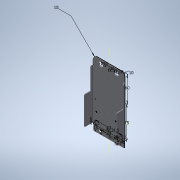
# Autodesk Inventor part: Enclosure_Base
Saved by Autodesk Inventor 2022 (Build 260153000, 153)
## iProperties
Created: 2023-10-31
Part Number: Enclosure_Base
Material: Generic
Document SubType Name: Sheet Metal
Designer: Baaij
Density: 1 g/cm^3
Sheet Metal Rule: Default_mm
Appearance: Default
Flat Pattern Width: 15 cm
Flat Pattern Length: 11.0786 cm
Flat Pattern Area: 166.179 cm^2
Sheet Metal Width: 150.000 mm
Sheet Metal Length: 110.786 mm
Sheet Metal Area: 16617.876 mm^2
Author: Baaij
Autodesk Inventor part; units mm, degrees
note: some values were not read from the file. Chosen so that the rebuilt part matches the saved one: relief shape of "Plate7"; flange form of "Plate6"; flange form of "Plate7"; relief shape of "Plate6".
ref_plane "YZ Plane" through (0, 0, 0) normal (1, 0, 0) x (0, 1, 0)
ref_plane "XZ Plane" through (0, 0, 0) normal (0, 1, 0) x (-1, 0, 0)
ref_plane "XY Plane" through (0, 0, 0) normal (0, 0, 1) x (1, 0, 0)
sketch "Sketch_base" plane through (0, 0, 0) normal (0, 0, 1) x (1, 0, 0)
  line L0 (0, 129.9853) -> (0, -82.9142) construction
  line L1 (-53.9995, 0) -> (53.9995, 0) construction
  line L2 (-36.5, 37.5) -> (36.5, 37.5)
  line L3 (36.5, 37.5) -> (36.5, -37.5)
  line L4 (36.5, -37.5) -> (-36.5, -37.5)
  line L5 (-36.5, -37.5) -> (-36.5, 37.5)
  line L6 (-36.5, 37.5) -> (36.5, -37.5) construction
  line L7 (36.5, 37.5) -> (-36.5, -37.5) construction
  line L8 (-35, -37.5) -> (35, -37.5)
  line L9 (35, -37.5) -> (35, -52.5)
  line L10 (35, -52.5) -> (-35, -52.5)
  line L11 (-35, -52.5) -> (-35, -37.5)
  line L12 (-35, -37.5) -> (35, -52.5) construction
  line L13 (35, -37.5) -> (-35, -52.5) construction
  line L14 (-26.5, 97.5) -> (26.5, 97.5)
  line L15 (36.5, 87.5) -> (36.5, 37.5)
  line L16 (36.5, 37.5) -> (-36.5, 37.5)
  line L17 (-36.5, 37.5) -> (-36.5, 87.5)
  line L18 (-36.5, 97.5) -> (36.5, 37.5) construction
  line L19 (36.5, 97.5) -> (-36.5, 37.5) construction
  arc A0 (-26.5, 97.5) -> (-36.5, 87.5) centre (-26.5, 87.5) ccw
  arc A1 (36.5, 87.5) -> (26.5, 97.5) centre (26.5, 87.5) ccw
  circle A2 centre (-30.5, 12.2) radius 1.6
  circle A3 centre (30.5, 12.2) radius 1.6
  circle A4 centre (16.2, -9.6) radius 2.5
  circle A5 centre (22.3, -9.6) radius 2.5
  circle A6 centre (28.6, -9.6) radius 2.5
  circle A7 centre (-31.5, -32) radius 1.6
  circle A8 centre (31.5, -32) radius 1.6
  circle A9 centre (-28, -12.5) radius 2.5
  point P0 (0, 0)
  point P1 (-20, -45.5)
  point P2 (20, -45.5)
  point P3 (0, -45)
  point P4 (0, 67.5)
  point P5 (-18, 87.5)
  point P6 (18, 87.5)
  point P7 (31.5, -32)
  dimension "d0" = 73
  dimension "d1" = 75
  dimension "d3" = 40
  dimension "d4" = 20
  dimension "d38" = 15
  dimension "d39" = 0
  dimension "d40" = 70
  dimension "d46" = 7
  dimension "d47" = 7
  dimension "d55" = 60
  dimension "d56" = 10
  dimension "d57" = 10
  dimension "d58" = 36
  dimension "d59" = 18
  dimension "d102" = 5.5
  dimension "d103" = 5.5
  dimension "d104" = 63
  dimension "d105" = 31.5
  dimension "d113" = 10
  dimension "d114" = 10
  constraints: 36 end point, 10 centre point, 6 midpoint, 6 parallel, 6 point on line, 4 point on circle, 4 tangent, 3 horizontal, 3 perpendicular, 16 other
  measures "d0" distance of L3.end L4.end
  measures "d1" distance of L2.end L3.end
  measures "d3" distance of point (20, -45.5) point (-20, -45.5)
  measures "d4" distance from line of L0 point (20, -45.5)
  measures "d38" distance between parallel lines of L8 L10
  measures "d39" distance between parallel lines of L4 L8
  measures "d40" distance between parallel lines of L9 L11
  measures "d46" distance from line of L10 point (-20, -45.5)
  measures "d47" distance from line of L10 point (20, -45.5)
  measures "d55" distance between parallel lines of L2 L14
  measures "d56" radius of A0
  measures "d57" radius of A1
  measures "d58" distance of point (18, 87.5) point (-18, 87.5)
  measures "d59" distance from line of L0 point (18, 87.5)
  measures "d102" distance from line of L8 point (-31.5, -32)
  measures "d103" distance from line of L8 point (31.5, -32)
  measures "d104" distance of point (31.5, -32) point (-31.5, -32)
  measures "d105" distance from line of L0 point (31.5, -32)
  measures "d113" distance from line of L14 point (-18, 87.5)
  measures "d114" distance from line of L14 point (18, 87.5)
extrude "Plate1" add sketch "Sketch_base" along normal blind 1.5 contours L2 L3 L4 L5 | A2 | A3 | A4 | A5 | A6 | A7 | A8 | A9
sheet face with bend "Face2" sketch "Sketch_base" thickness 1.5 toward (0, 0, 1) bend radius 1.5 contours L4 L9 L10 L11
bend "Bend3"
hole "Hole2" at (-20, -45.5, 0) at (20, -45.5, 0) direction (0, 0, 1) diameter 6 end through all
sheet face with bend "Face3" sketch "Sketch_base" thickness 1.5 toward (0, 0, 1) bend radius 1.5 contours L17 A0 L14 A1 L15 L2
bend "Bend4"
hole "Hole3" at (18, 87.5, 0) at (-18, 87.5, 0) direction (0, 0, 1) diameter 10 end through all
sketch "Sketch4" plane through (-36.5, -37.5, 1.5) normal (-1, 0, 0) x (0, -1, 0)
  line L0 (-115, 0) -> (0, 0)
  line L1 (0, 0) -> (0, 18.5)
  line L2 (0, 18.5) -> (-115, 18.5)
  line L3 (-115, 18.5) -> (-115, 0)
  constraints: 6 end point, 1 horizontal, 1 perpendicular, 1 vertical
edge flange "Flange3" height 20 angle 90 thickness 1.5 bend radius 1.5 thickness toward (-1, 0, 0) relief round relief width 1.5 relief depth 0.75 edges at (-36.5, 25, 1.5) wall of the first edge with corners at (-36.5, 77.5, 1.5) (-36.5, -37.5, 1.5) (-36.5, -37.5, 20) (-36.5, 77.5, 20)
bend "Bend5"
corner "Corner3"
sketch "Sketch5" plane through (36.5, 87.5, 1.5) normal (1, 0, 0) x (0, 1, 0)
  line L0 (-125, 0) -> (-10, 0)
  line L1 (-10, 0) -> (-10, 18.5)
  line L2 (-10, 18.5) -> (-125, 18.5)
  line L3 (-125, 18.5) -> (-125, 0)
  constraints: 8 end point
edge flange "Flange4" height 20 angle 90 thickness 1.5 bend radius 1.5 thickness toward (1, 0, 0) relief round relief width 1.5 relief depth 0.75 edges at (36.5, 25, 1.5) wall of the first edge with corners at (36.5, -37.5, 1.5) (36.5, 77.5, 1.5) (36.5, 77.5, 20) (36.5, -37.5, 20)
bend "Bend6"
corner "Corner4"
sketch "Sketch6" plane through (-38, -37.5, 20) normal (-1, 0, 0) x (0, 0, 1)
  line L0 (0, 0) -> (0, 115) projected
  line L1 (0, 115) -> (-15, 115)
  line L2 (-15, 115) -> (-15, 65)
  line L3 (-15, 65) -> (0, 65)
  line L4 (0, 65) -> (0, 115)
  point P0 (-20, 37.5)
  point P1 (0, 65)
  dimension "d96" = 15
  dimension "d97" = 50
  constraints: 8 end point, 2 parallel, 1 horizontal, 1 perpendicular
  measures "d96" distance of L3.end L2.end
  measures "d97" distance of L2.end L1.end
extrude "Extrusion1" cut sketch "Sketch6" against normal through all
fillet "Fillet1" radius 2 6 edges at (-37.25, 77.5, 5) (37.25, 77.5, 5) (37.25, 27.5, 20) (37.25, 27.5, 5) (-37.25, 27.5, 5) (-37.25, 27.5, 20)
fillet "Fillet2" radius 2 2 edges at (37.25, -37.5, 20) (-37.25, -37.5, 20)
hole "Hole4" at (-31.5, -32, 0) at (31.5, -32, 0) direction (0, 0, 1) diameter 3.2 end through all
fillet "Corner Round1" radius 2 2 edges at (-35, -52.5, 0.75) (35, -52.5, 0.75)
hole "Hole5" at (-30.5, 12.2, 0) at (30.5, 12.2, 0) direction (0, 0, 1) diameter 3.2 end through all
hole "Hole6" at (16.2, -9.6, 0) at (22.3, -9.6, 0) at (28.6, -9.6, 0) at (-28, -12.5, 0) direction (0, 0, 1) diameter 5 end through all
equation "\"d4\" = 0.5 * d3"
equation "\"d47\" = d46"
equation "\"d59\" = 0.5 * d58"
equation "\"d103\" = d102"
equation "\"d105\" = 0.5 * d104"
equation "\"d114\" = d113"
equation "\"d111\" = Thickness"
equation "\"d121\" = Thickness"
equation "\"d2\" = Thickness"
equation "\"d41\" = BendRadius"
equation "\"d42\" = BendReliefWidth"
equation "\"d44\" = MinimumRemnant"
equation "\"d43\" = BendReliefDepth"
equation "\"d45\" = TransitionRadius"
equation "\"d60\" = BendRadius"
equation "\"d61\" = BendReliefWidth"
equation "\"d63\" = MinimumRemnant"
equation "\"d62\" = BendReliefDepth"
equation "\"d64\" = TransitionRadius"
equation "\"d72\" = BendReliefWidth"
equation "\"d73\" = BendReliefDepth"
equation "\"d74\" = MinimumRemnant"
equation "\"d75\" = TransitionRadius"
equation "\"d78\" = BendRadius"
equation "\"d79\" = CornerReliefSize"
equation "\"d80\" = GapSize"
equation "\"d81\" = JacobiRadiusSize"
equation "\"d84\" = BendReliefWidth"
equation "\"d85\" = BendReliefDepth"
equation "\"d86\" = MinimumRemnant"
equation "\"d87\" = TransitionRadius"
equation "\"d92\" = BendRadius"
equation "\"d93\" = CornerReliefSize"
equation "\"d94\" = GapSize"
equation "\"d95\" = JacobiRadiusSize"
equation "\"BendRadius\" = Thickness"
equation "\"BendReliefWidth\" = Thickness"
equation "\"BendReliefDepth\" = 0.5 * Thickness"
equation "\"CornerReliefSize\" = 4 * Thickness"
equation "\"MinimumRemnant\" = 2 * Thickness"
equation "\"TransitionRadius\" = BendRadius"
equation "\"JacobiRadiusSize\" = BendRadius"
equation "\"GapSize\" = Thickness"
equation "\"Thickness\" = 1.5"
body "Solid1"
